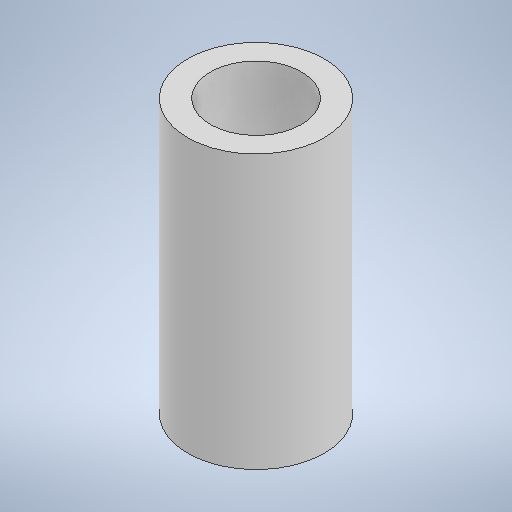
# Autodesk Inventor part: Part3
Saved by Autodesk Inventor 2025 (Build 290162000, 162)
## iProperties
Created: 2026-04-08
Part Number: Part3
Material: Generic
Document SubType Name: Modeling
Designer: lenovo
Density: 1 g/cm^3
Appearance: Default
Author: lenovo
Autodesk Inventor part; units mm, degrees
ref_plane "YZ Plane" through (0, 0, 0) normal (1, 0, 0) x (0, 1, 0)
ref_plane "XZ Plane" through (0, 0, 0) normal (0, 1, 0) x (-1, 0, 0)
ref_plane "XY Plane" through (0, 0, 0) normal (0, 0, 1) x (1, 0, 0)
sketch "Sketch1" plane through (0, 0, 0) normal (0, 0, 1) x (1, 0, 0)
  line L0 (0, 0) -> (5, 0) construction
  line L1 (5, 0) -> (7.5, 0)
  line L2 (0, 0) -> (0, 30) construction
  line L3 (5, 0) -> (5, 30)
  line L4 (5, 30) -> (0, 30) construction
  line L5 (7.5, 0) -> (7.5, 30)
  line L6 (7.5, 30) -> (5, 30)
  dimension "d1" = 2.5
  dimension "d2" = 5
  dimension "d3" = 30
  constraints: 14 end point, 3 vertical, 2 perpendicular, 1 horizontal, 1 point on line
  measures "d1" distance of L0.end L1.end
  measures "d2" distance of L0.start L0.end
  measures "d3" distance of L0.start L2.end
revolve "Revolution1" add sketch "Sketch1" angle 360 about axis through (0, 0, 0) along (0, 1, 0)
body "Solid1"
